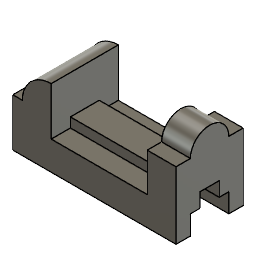
robocon_2 (Autodesk Fusion 360 design; units mm, degrees)
part number: 2026-03-05-17-14-59-870
part number: 2026-03-05-17-15-58-739
Autodesk Fusion 360 part; units mm, degrees
sketch "Sketch1" plane through (0, 0, 0) normal (1, 0, 0) x (0, 0, -1)
sketch "Sketch1 (2)" plane through (0, 0, 0) normal (0, 1, 0) x (1, 0, 0) in component "Component"
  line L0 (8.5, -3.5) -> (-8.5, -3.5)
  line L1 (-8.5, -3.5) -> (-8.5, 3.5)
  line L2 (-8.5, 3.5) -> (8.5, 3.5)
  line L3 (8.5, 3.5) -> (8.5, -3.5)
  line L4 (8.5, -3.5) -> (-8.5, 3.5) construction
  line L5 (-8.5, -3.5) -> (8.5, 3.5) construction
  dimension "d1" = 17
  dimension "d2" = 7
  constraint horizontal L0
  constraint perpendicular L0 L1
  constraint parallel L0 L2
  constraint parallel L1 L3
  constraint coincident L4 origin
  constraint coincident L5 origin
  measures "d1" distance of L1.end L2.end
  measures "d2" distance of L0.end L1.end
extrude "Extrude1" add sketch "Sketch1 (2)" along normal blind 5 in component "Component"
sketch "Sketch2" plane through (-8.5, 0, 0) normal (-1, 0, 0) x (0, 0, 1) in component "Component"
  line L0 (-3.5, 0) -> (3.5, 0)
  line L1 (3.5, 0) -> (3.5, 5)
  line L2 (3.5, 5) -> (-3.5, 5)
  line L3 (-3.5, 5) -> (-3.5, 0)
  line L4 (-2, 0) -> (-2, 2)
  line L5 (-2, 2) -> (-1, 2)
  line L6 (-1, 2) -> (-1, 3.5)
  line L7 (-1, 3.5) -> (1, 3.5)
  line L8 (1, 3.5) -> (1, 2)
  line L9 (1, 2) -> (2, 2)
  line L10 (2, 2) -> (2, 0)
  constraint coincident L0 L4.start
  constraint perpendicular L0 L4
  constraint perpendicular L4 L5
  constraint perpendicular L5 L6
  constraint perpendicular L6 L7
  constraint perpendicular L7 L8
  constraint perpendicular L8 L9
  constraint coincident L0 L10.end
  constraint perpendicular L0 L10
extrude "Extrude2" cut sketch "Sketch2" against normal up to surface (17 mm away) contours L0 L4 L5 L6 L7 L8 L9 L10 in component "Component"
sketch "Sketch3" plane through (0, 0, 3.5) normal (0, 0, 1) x (1, 0, 0) in component "Component"
  line L0 (-8.5, 0) -> (8.5, 0)
  line L1 (8.5, 0) -> (8.5, 5)
  line L2 (8.5, 5) -> (-8.5, 5)
  line L3 (-8.5, 5) -> (-8.5, 0)
  circle A0 centre (-4.5, 5) radius 3
  line L4 (-4.5, 5) -> (-4.5, 8)
  constraint coincident L2 A0.centre
  constraint coincident A0.centre L4.start
  constraint coincident A0 L4.end
  constraint perpendicular L2 L4
extrude "Extrude3" add sketch "Sketch3" against normal up to surface (7 mm away) contours L2 A0 L4 picked at (-5.6955, 6.597) in component "Component"
sketch "Sketch4" plane through (0, 5, 0) normal (0, 1, 0) x (-1, 0, 0) in component "Component"
  line L0 (4.5, -3.5) -> (4.5, 3.5)
  line L1 (4.5, 3.5) -> (-8.5, 3.5)
  line L2 (-8.5, 3.5) -> (-8.5, -3.5)
  line L3 (-8.5, -3.5) -> (4.5, -3.5)
  line L4 (-5.5, -3.5) -> (-5.5, 3.5)
  constraint coincident L3 L4.start
  constraint coincident L1 L4.end
  constraint perpendicular L1 L4
extrude "Extrude4" add sketch "Sketch4" along normal blind 2 contours L1 L2 L3 L4 in component "Component"
sketch "Sketch5" plane through (8.5, 0, 0) normal (1, 0, 0) x (0, 0, -1) in component "Component"
  line L0 (-2, 0) -> (-2, 2)
  line L1 (-2, 2) -> (-1, 2)
  line L2 (-1, 2) -> (-1, 3.5)
  line L3 (-1, 3.5) -> (1, 3.5)
  line L4 (1, 3.5) -> (1, 2)
  line L5 (1, 2) -> (2, 2)
  line L6 (2, 2) -> (2, 0)
  line L7 (2, 0) -> (3.5, 0)
  line L8 (3.5, 0) -> (3.5, 7)
  line L9 (3.5, 7) -> (-3.5, 7)
  line L10 (-3.5, 7) -> (-3.5, 0)
  line L11 (-3.5, 0) -> (-2, 0)
  circle A0 centre (0, 7) radius 2
  constraint midpoint L9 A0.centre
extrude "Extrude5" add sketch "Sketch5" against normal up to surface (3 mm away) contours L9 A0 picked at (0.4157, 7.5212) in component "Component"
sketch "Sketch6" plane through (0, 0, 3.5) normal (0, 0, 1) x (1, 0, 0) in component "Component"
  line L0 (-8.5, 0) -> (8.5, 0)
  line L1 (8.5, 0) -> (8.5, 7)
  line L2 (8.5, 7) -> (5.5, 7)
  line L3 (5.5, 7) -> (5.5, 5)
  line L4 (5.5, 5) -> (-4.5, 5)
  line L5 (-4.5, 5) -> (-4.5, 8)
  arc A0 (-4.5, 8) -> (-7.5, 5) centre (-4.5, 5) ccw
  line L6 (-7.5, 5) -> (-8.5, 5)
  line L7 (-8.5, 5) -> (-8.5, 0)
  line L8 (-4.5, 3) -> (5.5, 3)
  line L9 (5.5, 3) -> (5.5, 5)
  line L10 (-4.5, 3) -> (-4.5, 3.127)
  line L11 (-4.5, 3.127) -> (-4.5, 5)
  constraint parallel L0 L8
  constraint coincident L3.end L4.start
  constraint vertical L9
  constraint perpendicular L8 L10
  constraint coincident L4.end L5.start
  constraint parallel L5 L11
extrude "Extrude6" cut sketch "Sketch6" against normal blind 2 contours L4 L8 L9 L10 L11 in component "Component"
sketch "Sketch7" plane through (0, 0, -3.5) normal (0, 0, -1) x (-1, 0, 0) in component "Component"
  line L0 (-8.5, 0) -> (8.5, 0)
  line L1 (8.5, 0) -> (8.5, 5)
  line L2 (8.5, 5) -> (7.5, 5)
  arc A0 (7.5, 5) -> (4.5, 8) centre (4.5, 5) ccw
  line L3 (4.5, 8) -> (4.5, 5)
  line L4 (4.5, 5) -> (-5.5, 5)
  line L5 (-5.5, 5) -> (-5.5, 7)
  line L6 (-5.5, 7) -> (-8.5, 7)
  line L7 (-8.5, 7) -> (-8.5, 0)
  line L8 (-5.5, 3) -> (4.5, 3)
  line L9 (4.5, 3) -> (4.5, 5)
  line L10 (-5.5, 3) -> (-5.5, 5)
  constraint perpendicular L7 L8
  constraint coincident A0.centre L3.end
  constraint parallel L3 L9
  constraint coincident L4.end L5.start
  constraint parallel L5 L10
extrude "Extrude7" cut sketch "Sketch7" against normal blind 2 contours L4 L8 L9 L10 in component "Component"
sketch "Sketch8" plane through (0, 5, 0) normal (0, 1, 0) x (-1, 0, 0) in component "Component"
  line L0 (-5.5, -1.5) -> (4.5, -1.5)
  line L1 (4.5, -1.5) -> (4.5, 1.5)
  line L2 (4.5, 1.5) -> (-5.5, 1.5)
  line L3 (-5.5, 1.5) -> (-5.5, -1.5)
extrude "Extrude8" cut sketch "Sketch8" against normal blind 1 in component "Component"
component "Component" placed x (1, 0, 0) y (0, 1, 0) z (0, 0, 1) at (0, 0, 0)
